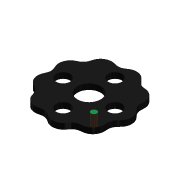
# Autodesk Inventor part: 180219-Disk
Saved by Autodesk Inventor 2022 (Build 260153000, 153)
## iProperties
Created: 2018-02-21
Part Number: 180219-Disk
Material: Bronze, Guss
Document SubType Name: Modeling
Designer: Normal
Mass: 138.711 g
Surface Area: 84.993 cm^2
Volume: 15.6382 cm^3
Density: 8.87 g/cm^3
Appearance: Bronze - satiniert
Author: Normal
Autodesk Inventor part; units mm, degrees
ref_plane "YZ Plane" through (0, 0, 0) normal (1, 0, 0) x (0, 1, 0)
ref_plane "XZ Plane" through (0, 0, 0) normal (0, 1, 0) x (-1, 0, 0)
ref_plane "XY Plane" through (0, 0, 0) normal (0, 0, 1) x (1, 0, 0)
derived "180219-Master.ipt"
sketch "Skizze2" plane through (0, 0, 0) normal (0, 0, 1) x (1, 0, 0)
  line L0 (0, 0) -> (9.3969, 3.4202) construction
  line L1 (0, 0) -> (9.3969, -3.4202) construction
  line L2 (0, 0) -> (42, 0) construction
  arc A0 (9.3969, -3.4202) -> (9.3969, 3.4202) centre (0, 0) ccw
  line L3 (9.3969, -3.4202) -> (31.0099, -11.2867)
  line L4 (9.3969, 3.4202) -> (31.0099, 11.2867)
  arc A1 (9.3969, 3.4202) -> (9.3969, -3.4202) centre (0, 0) ccw
  circle A2 centre (22.5, 0) radius 4
  circle A3 centre (22.5, 0) radius 6
  spline S0 degree 3 poles (31.0099, -11.2867) (31.0596, -11.15) (31.1671, -10.8796) (31.3182, -10.5552) (31.4787, -10.2448) (31.613, -10.0088) (31.785, -9.7307) (31.9245, -9.522) (32.1331, -9.2293) (32.3392, -8.963) (32.6366, -8.6062) (32.8861, -8.328) (33.1792, -8.0137) (33.4001, -7.7834) (33.6628, -7.5104) (33.8642, -7.3001) (34.1081, -7.0396) (34.2982, -6.8306) (34.5315, -6.5635) (34.7149, -6.3435) (34.9406, -6.0573) (35.1182, -5.8183) (35.3356, -5.505) (35.5054, -5.2423) (35.752, -4.8288) (35.9864, -4.3891) (36.3063, -3.681) (36.55, -3.0022) (36.7886, -2.1037) (36.9214, -1.3516) (37.0056, -0.3893) (37.0056, 0.3893) (36.9214, 1.3516) (36.7886, 2.1037) (36.55, 3.0022) (36.3063, 3.681) (35.9864, 4.3891) (35.752, 4.8288) (35.5054, 5.2423) (35.3356, 5.505) (35.1182, 5.8183) (34.9406, 6.0573) (34.7149, 6.3435) (34.5315, 6.5635) (34.2982, 6.8306) (34.1081, 7.0396) (33.8642, 7.3001) (33.6628, 7.5104) (33.4001, 7.7834) (33.1792, 8.0137) (32.8861, 8.328) (32.6366, 8.6062) (32.3392, 8.963) (32.1331, 9.2293) (31.9245, 9.522) (31.785, 9.7307) (31.613, 10.0088) (31.4787, 10.2448) (31.3182, 10.5552) (31.1671, 10.8796) (31.0596, 11.15) (31.0099, 11.2867) knots -0.349066 -0.349066 -0.349066 -0.349066 -0.341794 -0.334521 -0.330885 -0.323613 -0.319977 -0.312705 -0.309069 -0.29816 -0.290888 -0.276344 -0.269072 -0.254527 -0.247255 -0.232711 -0.225438 -0.210894 -0.203622 -0.189077 -0.181805 -0.167261 -0.159989 -0.145444 -0.138172 -0.116355 -0.101811 -0.072722 -0.058178 -0.029089 -0.014544 0.014544 0.029089 0.058178 0.072722 0.101811 0.116355 0.138172 0.145444 0.159989 0.167261 0.181805 0.189077 0.203622 0.210894 0.225438 0.232711 0.247255 0.254527 0.269072 0.276344 0.290888 0.29816 0.309069 0.312705 0.319977 0.323613 0.330885 0.334521 0.341794 0.349066 0.349066 0.349066 0.349066
  spline S1 degree 3 poles (35.7083, -12.9968) (35.9684, -12.2823) (36.5997, -11.6816) (37.4946, -10.7372) (38.384, -9.7987) (39.5052, -8.4934) (40.3973, -6.7316) (41.3238, -4.9021) (41.9604, -2.5931) (41.9981, -0.24) (42.0346, 2.0396) (41.5095, 4.3183) (40.6653, 6.1739) (39.8297, 8.0104) (38.7163, 9.4155) (37.7885, 10.423) (36.8593, 11.4319) (36.1466, 12.0655) (35.8121, 12.7523) (35.773, 12.8327) (35.7385, 12.9139) (35.7083, 12.9968) knots -0.349066 -0.349066 -0.349066 -0.349066 -0.235021 -0.235021 -0.235021 -0.121688 -0.121688 -0.121688 -0.004 -0.004 -0.004 0.110008 0.110008 0.110008 0.222841 0.222841 0.222841 0.335844 0.335844 0.335844 0.349066 0.349066 0.349066 0.349066
sketch "Skizze1" plane through (0, 0, 0) normal (0, 0, 1) x (1, 0, 0)
  circle A0 centre (0, 0) radius 40
  circle A1 centre (40, 0) radius 5
  line L0 (0, 0) -> (-2, 0)
  circle A2 centre (32.3607, 23.5114) radius 5
  circle A3 centre (12.3607, 38.0423) radius 5
  circle A4 centre (-12.3607, 38.0423) radius 5
  circle A5 centre (-32.3607, 23.5114) radius 5
  circle A6 centre (-40, 0) radius 5
  circle A7 centre (-32.3607, -23.5114) radius 5
  circle A8 centre (-12.3607, -38.0423) radius 5
  circle A9 centre (12.3607, -38.0423) radius 5
  circle A10 centre (32.3607, -23.5114) radius 5
  circle A11 centre (0, 0) radius 36
  circle A12 centre (40, 0) radius 4
  circle A13 centre (0, 0) radius 5
  circle A14 centre (-2, 0) radius 10
  point P0 (42, 0)
extrude "Extrusion1" add sketch "Skizze2" along normal blind 5 contours A0 L4 S0 L3 | A2 | A3
pattern_circular "Runde Anordnung1" count 9 over 360 about axis through (0, 0, -10) along (0, 0, 1)
extrude "Extrusion2" cut sketch "Skizze2" along normal through all contours A2 | A3
pattern_circular "Runde Anordnung2" count 4 over 360 about axis through (0, 0, -10) along (0, 0, 1) of "Extrusion2"
chamfer "Fase3" distance 0.1 angle 45 2 edges at (7.6604, -6.4279, 0) (-7.6604, 6.4279, 0)
sketch "草圖4" plane through (34.0049, 0, 5) normal (0, 0, 1) x (0.9396926, 0.3420201, 0)
  spline S0 degree 3 poles (1.1162, 10.6023) (1.1586, 10.2897) (1.2748, 9.7101) (1.5175, 8.9221) (1.7738, 8.2575) (2.0198, 7.6859) (2.2485, 7.1728) (2.46, 6.6889) (2.6557, 6.2123) (2.8358, 5.7273) (2.999, 5.2237) (3.142, 4.6949) (3.2606, 4.1379) (3.3501, 3.5521) (3.4054, 2.9392) (3.4221, 2.3027) (3.396, 1.6476) (3.3243, 0.98) (3.2049, 0.3067) (3.0373, -0.3648) (2.8221, -1.0271) (2.5612, -1.6729) (2.258, -2.2951) (1.9166, -2.8875) (1.5424, -3.4451) (1.1413, -3.9636) (0.7194, -4.4405) (0.2831, -4.8744) (-0.162, -5.2657) (-0.6109, -5.6161) (-1.0604, -5.9293) (-1.5091, -6.2102) (-1.9588, -6.4659) (-2.4151, -6.7053) (-2.8882, -6.94) (-3.3931, -7.1861) (-3.949, -7.4658) (-4.5725, -7.8101) (-5.2651, -8.2578) (-5.9948, -8.8425) (-6.693, -9.5663) (-7.2846, -10.3795) (-7.7337, -11.1997) (-8.0542, -11.9595) (-8.2851, -12.6333) (-8.464, -13.2293) (-8.6186, -13.7694) (-8.7677, -14.276) (-8.9242, -14.7669) (-9.0979, -15.2542) (-9.2967, -15.7449) (-9.527, -16.2419) (-9.7942, -16.7449) (-10.1022, -17.2511) (-10.4537, -17.7562) (-10.8501, -18.2544) (-11.2911, -18.7395) (-11.7752, -19.2048) (-12.2994, -19.6439) (-12.8595, -20.0506) (-13.4501, -20.4196) (-14.065, -20.7466) (-14.6973, -21.0283) (-15.3396, -21.2627) (-15.9846, -21.4493) (-16.6252, -21.5887) (-17.2549, -21.6828) (-17.8681, -21.7347) (-18.4605, -21.7484) (-19.0297, -21.7283) (-19.5753, -21.6793) (-20.0996, -21.6061) (-20.6085, -21.5128) (-21.1119, -21.4029) (-21.6251, -21.2787) (-22.1701, -21.1426) (-22.7757, -20.9995) (-23.4747, -20.8625) (-24.293, -20.7602) (-25.2278, -20.7391) (-26.2279, -20.8448) (-27.2039, -21.0875) (-28.0751, -21.4271) (-28.809, -21.8031) (-29.419, -22.1709) (-29.9392, -22.5125) (-30.4048, -22.8267) (-30.8446, -23.119) (-31.28, -23.3945) (-31.7263, -23.6562) (-32.194, -23.9043) (-32.6899, -24.1369) (-33.2179, -24.3505) (-33.7793, -24.5403) (-34.3732, -24.7012) (-34.9971, -24.8282) (-35.6468, -24.9163) (-36.3167, -24.9616) (-37.0005, -24.9609) (-37.6909, -24.9125) (-38.3806, -24.8155) (-39.0618, -24.6707) (-39.7272, -24.4801) (-40.3699, -24.2469) (-40.984, -23.9752) (-41.5643, -23.6702) (-42.1072, -23.3375) (-42.6103, -22.9832) (-43.0729, -22.6128) (-43.496, -22.2315) (-43.8824, -21.8433) (-44.237, -21.4502) (-44.5669, -21.0517) (-44.8819, -20.6439) (-45.1952, -20.2188) (-45.5252, -19.7642) (-45.8972, -19.2654) (-46.3446, -18.7111) (-46.9057, -18.1068) (-47.6082, -17.4897) (-48.4423, -16.9278) (-49.3459, -16.4864) (-50.2316, -16.1866) (-51.0355, -16.0028) (-51.7392, -15.8925) (-52.3572, -15.8198) (-52.9159, -15.7613) (-53.4407, -15.7024) (-53.9513, -15.6336) (-54.4614, -15.5472) (-54.9791, -15.4366) (-55.5086, -15.2961) (-56.0503, -15.1203) (-56.6023, -14.9048) (-57.1608, -14.6463) (-57.7203, -14.3425) (-58.2746, -13.9924) (-58.8169, -13.5965) (-59.3403, -13.1565) (-59.8381, -12.6755) (-60.304, -12.158) (-60.7328, -11.6092) (-61.12, -11.0355) (-61.4625, -10.4436) (-61.7582, -9.8408) (-62.0067, -9.2341) (-62.2088, -8.6304) (-62.3664, -8.0355) (-62.4827, -7.4545) (-62.5617, -6.8904) (-62.6082, -6.3446) (-62.6271, -5.8155) (-62.6237, -5.2982) (-62.6028, -4.7834) (-62.5696, -4.2563) (-62.5302, -3.696) (-62.4945, -3.0748) (-62.481, -2.3626) (-62.5224, -1.539) (-62.6638, -0.6147) (-62.9417, 0.3519) (-63.3501, 1.2708) (-63.8359, 2.0699) (-64.3336, 2.7274) (-64.8017, 3.2642) (-65.2284, 3.7171) (-65.6188, 4.1211) (-65.983, 4.5035) (-66.3299, 4.8844) (-66.6651, 5.2785) (-66.9906, 5.696) (-67.3059, 6.144) (-67.6079, 6.6269) (-67.8923, 7.1467) (-68.1539, 7.7037) (-68.3872, 8.2961) (-68.5868, 8.9206) (-68.7477, 9.5725) (-68.8658, 10.246) (-68.938, 10.9344) (-68.9623, 11.6304) (-68.938, 12.3264) (-68.8658, 13.0147) (-68.7477, 13.6882) (-68.5868, 14.3401) (-68.3872, 14.9646) (-68.1539, 15.557) (-67.8923, 16.114) (-67.6079, 16.6339) (-67.3059, 17.1167) (-66.9906, 17.5647) (-66.6651, 17.9822) (-66.3299, 18.3763) (-65.983, 18.7573) (-65.6188, 19.1397) (-65.2284, 19.5436) (-64.8017, 19.9966) (-64.3336, 20.5334) (-63.8359, 21.1909) (-63.3501, 21.9899) (-62.9417, 22.9089) (-62.6638, 23.8754) (-62.5224, 24.7997) (-62.481, 25.6233) (-62.4945, 26.3355) (-62.5302, 26.9567) (-62.5696, 27.5171) (-62.6028, 28.0441) (-62.6237, 28.559) (-62.6271, 29.0763) (-62.6082, 29.6054) (-62.5617, 30.1512) (-62.4827, 30.7152) (-62.3664, 31.2963) (-62.2088, 31.8911) (-62.0067, 32.4949) (-61.7582, 33.1016) (-61.4625, 33.7044) (-61.12, 34.2962) (-60.7328, 34.87) (-60.304, 35.4187) (-59.8381, 35.9363) (-59.3403, 36.4172) (-58.8169, 36.8572) (-58.2746, 37.2532) (-57.7203, 37.6033) (-57.1608, 37.9071) (-56.6023, 38.1656) (-56.0503, 38.381) (-55.5086, 38.5568) (-54.9791, 38.6973) (-54.4614, 38.8079) (-53.9513, 38.8943) (-53.4407, 38.9632) (-52.9159, 39.022) (-52.3572, 39.0805) (-51.7392, 39.1532) (-51.0355, 39.2635) (-50.2316, 39.4473) (-49.3459, 39.7472) (-48.4423, 40.1886) (-47.6082, 40.7504) (-46.9057, 41.3675) (-46.3446, 41.9719) (-45.8972, 42.5261) (-45.5252, 43.025) (-45.1952, 43.4795) (-44.8819, 43.9046) (-44.5669, 44.3124) (-44.237, 44.7109) (-43.8824, 45.104) (-43.496, 45.4923) (-43.0729, 45.8735) (-42.6103, 46.2439) (-42.1072, 46.5983) (-41.5643, 46.9309) (-40.984, 47.2359) (-40.3699, 47.5076) (-39.7272, 47.7409) (-39.0618, 47.9315) (-38.3806, 48.0762) (-37.6909, 48.1732) (-37.0005, 48.2217) (-36.3167, 48.2223) (-35.6468, 48.177) (-34.9971, 48.0889) (-34.3732, 47.962) (-33.7793, 47.8011) (-33.2179, 47.6112) (-32.6899, 47.3977) (-32.194, 47.165) (-31.7263, 46.9169) (-31.28, 46.6552) (-30.8446, 46.3798) (-30.4048, 46.0875) (-29.9392, 45.7732) (-29.419, 45.4317) (-28.809, 45.0638) (-28.0751, 44.6879) (-27.2039, 44.3482) (-26.2279, 44.1056) (-25.2278, 43.9998) (-24.293, 44.021) (-23.4747, 44.1233) (-22.7757, 44.2603) (-22.1701, 44.4033) (-21.6251, 44.5394) (-21.1119, 44.6636) (-20.6085, 44.7736) (-20.0996, 44.8668) (-19.5753, 44.94) (-19.0297, 44.989) (-18.4605, 45.0091) (-17.8681, 44.9955) (-17.2549, 44.9436) (-16.6252, 44.8494) (-15.9846, 44.71) (-15.3396, 44.5235) (-14.6973, 44.289) (-14.065, 44.0073) (-13.4501, 43.6803) (-12.8595, 43.3113) (-12.2994, 42.9046) (-11.7752, 42.4656) (-11.2911, 42.0003) (-10.8501, 41.5152) (-10.4537, 41.0169) (-10.1022, 40.5119) (-9.7942, 40.0056) (-9.527, 39.5026) (-9.2967, 39.0056) (-9.0979, 38.5149) (-8.9242, 38.0276) (-8.7677, 37.5367) (-8.6186, 37.0301) (-8.464, 36.4901) (-8.2851, 35.8941) (-8.0542, 35.2202) (-7.7337, 34.4605) (-7.2846, 33.6403) (-6.693, 32.8271) (-5.9948, 32.1032) (-5.2651, 31.5185) (-4.5725, 31.0709) (-3.949, 30.7265) (-3.3931, 30.4468) (-2.8882, 30.2008) (-2.4151, 29.966) (-1.9588, 29.7267) (-1.5091, 29.471) (-1.0604, 29.19) (-0.6109, 28.8769) (-0.162, 28.5264) (0.2831, 28.1352) (0.7194, 27.7012) (1.1413, 27.2244) (1.5424, 26.7058) (1.9166, 26.1483) (2.258, 25.5558) (2.5612, 24.9336) (2.8221, 24.2879) (3.0373, 23.6256) (3.2049, 22.954) (3.3243, 22.2807) (3.396, 21.6131) (3.4221, 20.958) (3.4054, 20.3216) (3.3501, 19.7087) (3.2606, 19.1229) (3.142, 18.5659) (2.999, 18.0371) (2.8358, 17.5334) (2.6557, 17.0484) (2.46, 16.5718) (2.2485, 16.0879) (2.0198, 15.5748) (1.7738, 15.0033) (1.5175, 14.3387) (1.2747, 13.5506) (1.0916, 12.6336) (1.0218, 11.6305) (1.07, 10.9427) (1.1162, 10.6023) knots 0 0 0 0 0.004014 0.007499 0.010478 0.013071 0.015414 0.017624 0.019788 0.021968 0.024203 0.026521 0.028933 0.031445 0.034054 0.036756 0.039538 0.042388 0.045291 0.048229 0.051186 0.054143 0.057081 0.059984 0.062834 0.065617 0.068318 0.070928 0.07344 0.075852 0.078169 0.080405 0.082584 0.084748 0.086958 0.089302 0.091894 0.094873 0.098359 0.102372 0.106742 0.111111 0.115125 0.11861 0.121589 0.124182 0.126525 0.128735 0.130899 0.133079 0.135315 0.137632 0.140044 0.142556 0.145166 0.147867 0.150649 0.153499 0.156402 0.159341 0.162297 0.165254 0.168192 0.171095 0.173945 0.176728 0.179429 0.182039 0.184551 0.186963 0.18928 0.191516 0.193695 0.195859 0.198069 0.200413 0.203006 0.205984 0.20947 0.213483 0.217853 0.222222 0.226236 0.229721 0.2327 0.235293 0.237636 0.239846 0.24201 0.24419 0.246426 0.248743 0.251155 0.253667 0.256277 0.258978 0.26176 0.26461 0.267513 0.270452 0.273408 0.276365 0.279304 0.282206 0.285056 0.287839 0.29054 0.29315 0.295662 0.298074 0.300391 0.302627 0.304806 0.306971 0.309181 0.311524 0.314117 0.317096 0.320581 0.324594 0.328964 0.333333 0.337347 0.340832 0.343811 0.346404 0.348747 0.350957 0.353121 0.355301 0.357537 0.359854 0.362266 0.364778 0.367388 0.370089 0.372871 0.375722 0.378624 0.381563 0.384519 0.387476 0.390415 0.393317 0.396168 0.39895 0.401651 0.404261 0.406773 0.409185 0.411502 0.413738 0.415918 0.418082 0.420292 0.422635 0.425228 0.428207 0.431692 0.435706 0.440075 0.444444 0.448458 0.451943 0.454922 0.457515 0.459858 0.462068 0.464232 0.466412 0.468648 0.470965 0.473377 0.475889 0.478499 0.4812 0.483982 0.486833 0.489735 0.492674 0.495631 0.498587 0.501526 0.504428 0.507279 0.510061 0.512762 0.515372 0.517884 0.520296 0.522613 0.524849 0.527029 0.529193 0.531403 0.533746 0.536339 0.539318 0.542803 0.546817 0.551186 0.555556 0.559569 0.563054 0.566033 0.568626 0.570969 0.573179 0.575344 0.577523 0.579759 0.582076 0.584488 0.587 0.58961 0.592311 0.595094 0.597944 0.600846 0.603785 0.606742 0.609698 0.612637 0.61554 0.61839 0.621172 0.623873 0.626483 0.628995 0.631407 0.633724 0.63596 0.63814 0.640304 0.642514 0.644857 0.64745 0.650429 0.653914 0.657928 0.662297 0.666667 0.67068 0.674166 0.677144 0.679737 0.682081 0.684291 0.686455 0.688634 0.69087 0.693187 0.695599 0.698111 0.700721 0.703422 0.706205 0.709055 0.711958 0.714896 0.717853 0.720809 0.723748 0.726651 0.729501 0.732283 0.734984 0.737594 0.740106 0.742518 0.744835 0.747071 0.749251 0.751415 0.753625 0.755968 0.758561 0.76154 0.765025 0.769039 0.773408 0.777778 0.781791 0.785277 0.788256 0.790848 0.793192 0.795402 0.797566 0.799745 0.801981 0.804298 0.80671 0.809222 0.811832 0.814533 0.817316 0.820166 0.823069 0.826007 0.828964 0.831921 0.834859 0.837762 0.840612 0.843394 0.846096 0.848705 0.851217 0.853629 0.855947 0.858182 0.860362 0.862526 0.864736 0.867079 0.869672 0.872651 0.876136 0.88015 0.884519 0.888889 0.892902 0.896388 0.899367 0.901959 0.904303 0.906513 0.908677 0.910856 0.913092 0.915409 0.917822 0.920333 0.922943 0.925645 0.928427 0.931277 0.93418 0.937118 0.940075 0.943032 0.94597 0.948873 0.951723 0.954505 0.957207 0.959817 0.962328 0.964741 0.967058 0.969294 0.971473 0.973637 0.975847 0.978191 0.980783 0.983762 0.987248 0.991261 0.995631 1 1 1 1
  point P0 (-31.9542, 11.6304)
  point P1 (1.5389, 8.8874)
  point P2 (1.7892, 8.231)
  point P3 (2.0288, 7.6685)
  point P4 (2.2521, 7.163)
  point P5 (2.4596, 6.6849)
  point P6 (2.6525, 6.2124)
  point P7 (2.8309, 5.7303)
  point P8 (2.9929, 5.2285)
  point P9 (3.1353, 4.7009)
  point P10 (3.2536, 4.1445)
  point P11 (3.343, 3.559)
  point P12 (3.3983, 2.946)
  point P13 (3.415, 2.3091)
  point P14 (3.389, 1.6535)
  point P15 (3.3172, 0.9852)
  point P16 (3.1977, 0.3111)
  point P17 (3.0299, -0.3612)
  point P18 (2.8144, -1.0244)
  point P19 (2.5533, -1.6709)
  point P20 (2.2496, -2.2938)
  point P21 (1.9079, -2.887)
  point P22 (1.5333, -3.445)
  point P23 (1.1318, -3.964)
  point P24 (0.7097, -4.4411)
  point P25 (0.2732, -4.8751)
  point P26 (-0.1716, -5.2663)
  point P27 (-0.6199, -5.6165)
  point P28 (-1.0681, -5.9291)
  point P29 (-1.5148, -6.2093)
  point P30 (-1.9613, -6.464)
  point P31 (-2.4128, -6.7019)
  point P32 (-2.879, -6.9348)
  point P33 (-3.375, -7.1785)
  point P34 (-3.9202, -7.4554)
  point P35 (-4.5339, -7.7973)
  point P36 (-5.2227, -8.2458)
  point P37 (-5.96, -8.8393)
  point P38 (-6.6747, -9.5816)
  point P39 (-7.2816, -10.4144)
  point P40 (-7.7381, -11.2435)
  point P41 (-8.0601, -11.9998)
  point P42 (-8.2903, -12.6635)
  point P43 (-8.4683, -13.2485)
  point P44 (-8.6222, -13.7792)
  point P45 (-8.7706, -14.2789)
  point P46 (-8.9265, -14.7648)
  point P47 (-9.0998, -15.2488)
  point P48 (-9.2981, -15.7373)
  point P49 (-9.5282, -16.233)
  point P50 (-9.7952, -16.7353)
  point P51 (-10.1032, -17.2413)
  point P52 (-10.4548, -17.7464)
  point P53 (-10.8514, -18.245)
  point P54 (-11.2928, -18.7305)
  point P55 (-11.7773, -19.1963)
  point P56 (-12.3021, -19.6359)
  point P57 (-12.8628, -20.0431)
  point P58 (-13.4542, -20.4126)
  point P59 (-14.0698, -20.7399)
  point P60 (-14.7028, -21.022)
  point P61 (-15.3459, -21.2566)
  point P62 (-15.9916, -21.4434)
  point P63 (-16.6328, -21.5829)
  point P64 (-17.2628, -21.677)
  point P65 (-17.8761, -21.729)
  point P66 (-18.4683, -21.7427)
  point P67 (-19.0368, -21.7228)
  point P68 (-19.5811, -21.6742)
  point P69 (-20.1034, -21.6017)
  point P70 (-20.6091, -21.5098)
  point P71 (-21.1079, -21.4018)
  point P72 (-21.6148, -21.2805)
  point P73 (-22.1514, -21.1484)
  point P74 (-22.747, -21.0101)
  point P75 (-23.4369, -20.8775)
  point P76 (-24.2528, -20.7783)
  point P77 (-25.1991, -20.7591)
  point P78 (-26.2238, -20.8683)
  point P79 (-27.224, -21.1161)
  point P80 (-28.1067, -21.4579)
  point P81 (-28.8394, -21.8302)
  point P82 (-29.4424, -22.1906)
  point P83 (-29.9548, -22.5244)
  point P84 (-30.4138, -22.832)
  point P85 (-30.8487, -23.1194)
  point P86 (-31.2805, -23.3914)
  point P87 (-31.7243, -23.6508)
  point P88 (-32.1902, -23.8975)
  point P89 (-32.6851, -24.1293)
  point P90 (-33.2125, -24.3425)
  point P91 (-33.7737, -24.5321)
  point P92 (-34.3678, -24.6931)
  point P93 (-34.992, -24.8201)
  point P94 (-35.6422, -24.9083)
  point P95 (-36.3128, -24.9537)
  point P96 (-36.9974, -24.9531)
  point P97 (-37.6887, -24.9046)
  point P98 (-38.3792, -24.8075)
  point P99 (-39.0612, -24.6626)
  point P100 (-39.7274, -24.4717)
  point P101 (-40.3709, -24.2381)
  point P102 (-40.9855, -23.9661)
  point P103 (-41.5663, -23.6609)
  point P104 (-42.1095, -23.328)
  point P105 (-42.6127, -22.9736)
  point P106 (-43.0752, -22.6034)
  point P107 (-43.4979, -22.2227)
  point P108 (-43.8836, -21.8356)
  point P109 (-44.2371, -21.4444)
  point P110 (-44.5654, -21.0489)
  point P111 (-44.8781, -20.6456)
  point P112 (-45.1885, -20.2269)
  point P113 (-45.5146, -19.7807)
  point P114 (-45.8819, -19.2919)
  point P115 (-46.3252, -18.7469)
  point P116 (-46.8865, -18.1465)
  point P117 (-47.5991, -17.5234)
  point P118 (-48.4542, -16.9485)
  point P119 (-49.3797, -16.4954)
  point P120 (-50.2755, -16.1898)
  point P121 (-51.0762, -16.004)
  point P122 (-51.7698, -15.8926)
  point P123 (-52.3768, -15.8188)
  point P124 (-52.9262, -15.7595)
  point P125 (-53.444, -15.7001)
  point P126 (-53.9497, -15.6309)
  point P127 (-54.4563, -15.5444)
  point P128 (-54.9719, -15.4338)
  point P129 (-55.5, -15.2933)
  point P130 (-56.041, -15.1176)
  point P131 (-56.5928, -14.9022)
  point P132 (-57.1514, -14.6436)
  point P133 (-57.7112, -14.3396)
  point P134 (-58.266, -13.9893)
  point P135 (-58.8089, -13.593)
  point P136 (-59.3329, -13.1525)
  point P137 (-59.8313, -12.671)
  point P138 (-60.2978, -12.1528)
  point P139 (-60.7271, -11.6033)
  point P140 (-61.1148, -11.0289)
  point P141 (-61.4576, -10.4364)
  point P142 (-61.7536, -9.8329)
  point P143 (-62.0023, -9.2257)
  point P144 (-62.2044, -8.6216)
  point P145 (-62.3621, -8.0266)
  point P146 (-62.4784, -7.4458)
  point P147 (-62.5575, -6.8825)
  point P148 (-62.6042, -6.338)
  point P149 (-62.6235, -5.8111)
  point P150 (-62.6208, -5.2971)
  point P151 (-62.6011, -4.7871)
  point P152 (-62.5697, -4.2669)
  point P153 (-62.5327, -3.7155)
  point P154 (-62.4999, -3.1049)
  point P155 (-62.4892, -2.4025)
  point P156 (-62.5332, -1.5817)
  point P157 (-62.6786, -0.6464)
  point P158 (-62.964, 0.3437)
  point P159 (-63.3818, 1.2857)
  point P160 (-63.8716, 2.0956)
  point P161 (-64.3655, 2.7526)
  point P162 (-64.8252, 3.2838)
  point P163 (-65.2428, 3.7304)
  point P164 (-65.6256, 4.1291)
  point P165 (-65.984, 4.5074)
  point P166 (-66.3269, 4.8854)
  point P167 (-66.6594, 5.2774)
  point P168 (-66.9833, 5.6935)
  point P169 (-67.2975, 6.1406)
  point P170 (-67.599, 6.623)
  point P171 (-67.8833, 7.1427)
  point P172 (-68.1449, 7.6998)
  point P173 (-68.3784, 8.2925)
  point P174 (-68.5782, 8.9175)
  point P175 (-68.7393, 9.5701)
  point P176 (-68.8576, 10.2443)
  point P177 (-68.9299, 10.9335)
  point P178 (-68.9542, 11.6304)
  point P179 (-68.9299, 12.3272)
  point P180 (-68.8576, 13.0164)
  point P181 (-68.7393, 13.6907)
  point P182 (-68.5782, 14.3432)
  point P183 (-68.3784, 14.9682)
  point P184 (-68.1449, 15.561)
  point P185 (-67.8833, 16.1181)
  point P186 (-67.599, 16.6378)
  point P187 (-67.2975, 17.1202)
  point P188 (-66.9833, 17.5672)
  point P189 (-66.6594, 17.9833)
  point P190 (-66.3269, 18.3753)
  point P191 (-65.984, 18.7533)
  point P192 (-65.6256, 19.1317)
  point P193 (-65.2428, 19.5303)
  point P194 (-64.8252, 19.9769)
  point P195 (-64.3655, 20.5081)
  point P196 (-63.8716, 21.1651)
  point P197 (-63.3818, 21.9751)
  point P198 (-62.964, 22.917)
  point P199 (-62.6786, 23.9071)
  constraints: 360 other
sketch "草圖5" plane through (34.0049, 0, 5) normal (0, 0, 1) x (0.9396926, 0.3420201, 0)
  circle A0 centre (-14.7042, -18.2475) radius 2.5
  line L0 (-26.2238, -20.8683) -> (-14.7042, -18.2475)
  line L1 (-14.7042, -18.2475) -> (-6.6747, -9.5816)
  point P0 (-31.9542, 11.6304)
  dimension "d20" = 5
  constraints: 4 end point, 1 centre point, 1 equal length, 2 other
  measures "d20" diameter of A0
extrude "擠出3" add sketch "草圖5" along normal blind 10
